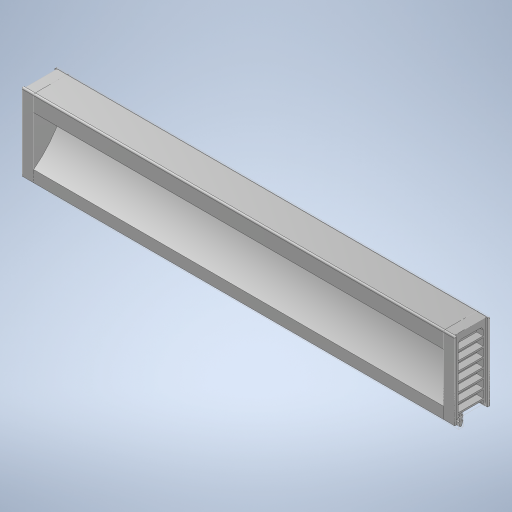
# Autodesk Inventor part: Hafele_alu_126_39
Saved by Autodesk Inventor 2024 (Build 280153000, 153)
## iProperties
RuleStatus: InUse
Created: 2019-10-04
Part Number: Hafele_alu_126_39
Material: Aluminum 6061
Document SubType Name: Modeling
Designer: RokasM
Density: 2.7 g/cm^3
Appearance: Anodized - Light Gray
AfterDocOpen0: LengthRule
Author: RokasM
Autodesk Inventor part; units mm, degrees
ref_plane "XZ Plane" through (0, 0, 0) normal (0, 1, 0) x (-1, 0, 0)
ref_plane "XY Plane" through (0, 0, 0) normal (0, 0, 1) x (1, 0, 0)
sketch "Sketch1" plane through (0, 0, 0) normal (1, 0, 0) x (0, 1, 0)
  line L0 (19.2576, 47.182) -> (19.2576, 36.782)
  line L1 (19.2576, 36.782) -> (21.0176, 36.782)
  arc A0 (24.8576, 45.482) -> (21.0176, 36.782) centre (44.137, 31.775) ccw
  line L2 (24.8576, 45.482) -> (38.8576, 45.482)
  line L3 (38.8576, 45.482) -> (38.8576, 34.7948)
  arc A1 (38.8223, 34.5717) -> (38.8576, 34.7948) centre (38.1341, 34.7948) ccw
  arc A2 (19.2576, 7.182) -> (38.8223, 34.5717) centre (-14.1874, 51.7546) ccw
  line L4 (19.2576, 7.182) -> (19.2576, 0.182)
  line L5 (19.2576, 0.182) -> (20.2576, 0.182)
  line L6 (20.2576, 0.182) -> (20.2576, 2.182)
  line L7 (20.2576, 2.182) -> (29.4376, 2.182)
  line L8 (29.4376, 2.182) -> (29.4376, -0.568)
  line L9 (29.4376, -0.568) -> (28.5076, -0.568)
  line L10 (28.5076, -0.568) -> (29.4376, -3.318)
  line L11 (29.4376, -3.318) -> (28.5076, -3.318)
  line L12 (28.5076, -3.318) -> (29.4376, -6.068)
  line L13 (29.4376, -6.068) -> (28.5076, -6.068)
  line L14 (28.5076, -6.068) -> (29.4376, -8.818)
  line L15 (29.4376, -8.818) -> (30.3776, -8.818)
  line L16 (30.3776, -8.818) -> (31.3076, -6.068)
  line L17 (31.3076, -6.068) -> (30.3776, -6.068)
  line L18 (30.3776, -6.068) -> (31.3076, -3.318)
  line L19 (31.3076, -3.318) -> (30.3776, -3.318)
  line L20 (30.3776, -3.318) -> (31.3076, -0.568)
  line L21 (31.3076, -0.568) -> (30.3776, -0.568)
  line L22 (30.3776, -0.568) -> (30.3776, 2.182)
  line L23 (30.3776, 2.182) -> (38.8576, 2.182)
  line L24 (38.8576, 2.182) -> (38.8576, 0.182)
  line L25 (38.8576, 0.182) -> (40.5576, 0.182)
  line L26 (40.5576, 0.182) -> (40.5576, 47.182)
  line L27 (40.5576, 47.182) -> (19.2576, 47.182)
  line L28 (21.6706, 3.882) -> (21.6706, 6.901)
  arc A3 (21.6706, 6.901) -> (38.8576, 29.7576) centre (-14.1874, 51.7546) ccw
  line L29 (38.8576, 29.7576) -> (38.8576, 3.882)
  line L30 (38.8576, 3.882) -> (21.6706, 3.882)
  point P0 (0, 0)
  dimension "d0" = 21.3
  dimension "d1" = 45
  dimension "d2" = 2
  dimension "d3" = 1
  dimension "d4" = 1.7
  dimension "d5" = 10.4
  dimension "d6" = 7
  dimension "d7" = 2.8
  dimension "d8" = 56
  dimension "d9" = 0.93
  dimension "d10" = 2.75
  dimension "d11" = 10.18
  dimension "d12" = 1.7
  dimension "d13" = 1.7
  dimension "d14" = 1.76
  dimension "d16" = 14
  dimension "d17" = 15.407
  dimension "d22" = 55.725
  dimension "d26" = 57.425
  dimension "d28" = 1.7
  dimension "d29" = 10.9103
  dimension "d30" = 2.413
  dimension "d31" = 1.7
  constraints: 62 end point, 10 horizontal, 9 vertical, 8 point on circle, 6 collinear, 6 vertical alignment, 5 equal length, 4 centre point, 4 parallel, 2 tangent, 1 concentric
  measures "d0" distance between parallel lines of L26 L0
  measures "d1" distance between parallel lines of L23 L27
  measures "d2" distance between parallel lines of L7 L5
  measures "d3" distance between parallel lines of L4 L6
  measures "d4" distance between parallel lines of L26 L24
  measures "d5" distance between parallel lines of L1 L27
  measures "d6" distance of L4.start L4.end
  measures "d7" distance of L16.end L13.end
  measures "d8" distance between parallel lines of L27 L15
  measures "d9" distance of L8.end L9.end
  measures "d10" distance between parallel lines of L11 L9
  measures "d11" distance between parallel lines of L8 L4
  measures "d12" distance between parallel lines of L2 L27
  measures "d13" distance between parallel lines of L26 L3
  measures "d14" distance of L0.end L1.end
  measures "d16" distance from line of L2.start L3
  measures "d17" distance from line of A0.centre L27
  measures "d22" radius of A2
  measures "d26" radius of A3
  measures "d28" distance between parallel lines of L26 L29
  measures "d29" distance from line of L2 A1.start
  measures "d30" distance between parallel lines of L4 L28
  measures "d31" distance between parallel lines of L7 L30
extrude "01_ex1" add sketch "Sketch1" along normal mid plane 250
fillet "01_fillet" radius 1.5 1 edges at (0, 38.8576, 29.7576)
fillet "01_fillet" radius 1 4 edges at (0, 21.0176, 36.782) (0, 19.2576, 47.182) (0, 38.8576, 45.482) (0, 40.5576, 47.182)
fillet "01_fillet" radius 0.5 6 edges at (0, 19.2576, 36.782) (0, 24.8576, 45.482) (0, 38.8576, 3.882) (0, 21.6706, 3.882) (0, 21.6706, 6.901) (0, 20.2576, 2.182)
ref_plane "wp_right" through (125, 0, 0) normal (1, 0, 0) x (0, 1, 0)
sketch "Sketch2" plane through (125, 0, 0) normal (1, 0, 0) x (0, 1, 0)
  line L0 (19.2576, 47.182) -> (40.5576, 47.182)
  line L1 (40.5576, 47.182) -> (40.5576, 0.182)
  line L2 (40.5576, 0.182) -> (19.2576, 0.182)
  line L3 (19.2576, 0.182) -> (19.2576, 47.182)
  line L4 (39.5576, 47.182) -> (20.2576, 47.182) projected
  line L5 (40.5576, 0.182) -> (40.5576, 46.182) projected
  point P0 (0, 0)
  dimension "d38" = 21.3
  dimension "d39" = 47
  constraints: 8 end point, 2 collinear, 2 parallel, 1 horizontal, 1 perpendicular
  measures "d38" distance between parallel lines of L1 L3
  measures "d39" distance between parallel lines of L2 L0
extrude "02_ex1" add sketch "Sketch2" along normal blind 7 separate body
sketch "Sketch3" plane through (132, 0, 0) normal (1, 0, 0) x (0, 0, -1)
  line L0 (-47.182, 20.2576) -> (-0.182, 20.2576)
  line L1 (-0.182, 20.2576) -> (-0.182, 39.1576)
  line L2 (-0.182, 39.1576) -> (-47.182, 39.1576)
  line L3 (-47.182, 39.1576) -> (-47.182, 20.2576)
  line L4 (-47.182, 19.2576) -> (-0.182, 19.2576) projected
  line L5 (-0.182, 19.2576) -> (-0.182, 40.5576) projected
  line L6 (-47.182, 40.5576) -> (-47.182, 19.2576) projected
  point P0 (0, 0)
  dimension "d42" = 18.9
  dimension "d43" = 1
  constraints: 8 end point, 2 collinear, 2 parallel, 1 horizontal, 1 perpendicular
  measures "d42" distance between parallel lines of L2 L0
  measures "d43" distance between parallel lines of L4 L0
extrude "02_ex2" cut sketch "Sketch3" against normal blind 1 contours L3 L2 L1 L0 bodies 2
sketch "Sketch4" plane through (131, 0, 0) normal (1, 0, 0) x (0, 0, -1)
  line L0 (-2.182, 39.1576) -> (-0.182, 39.1576)
  line L1 (-0.182, 39.1576) -> (-0.182, 20.2576)
  line L2 (-0.182, 20.2576) -> (-2.182, 20.2576)
  line L3 (-2.182, 20.2576) -> (-2.182, 39.1576)
  line L4 (-47.182, 39.1576) -> (-0.182, 39.1576) projected
  line L5 (-0.182, 20.2576) -> (-47.182, 20.2576) projected
  line L6 (-0.182, 39.1576) -> (-0.182, 20.2576) projected
  point P0 (0, 0)
  dimension "d46" = 2
  constraints: 8 end point, 3 collinear, 2 parallel, 1 horizontal, 1 perpendicular
  measures "d46" distance between parallel lines of L1 L3
extrude "02_ex3" cut sketch "Sketch4" against normal up to surface (6 mm away) bodies 2
sketch "Sketch5" plane through (131, 0, 0) normal (1, 0, 0) x (0, 0, -1)
  line L0 (-43.182, 22.2576) -> (-2.182, 22.2576)
  line L1 (-2.182, 22.2576) -> (-2.182, 37.5576)
  line L2 (-2.182, 37.5576) -> (-43.182, 37.5576)
  line L3 (-43.182, 37.5576) -> (-43.182, 22.2576)
  line L4 (-0.182, 20.2576) -> (-47.182, 20.2576) projected
  line L5 (-2.182, 20.2576) -> (-2.182, 39.1576) projected
  point P0 (0, 0)
  dimension "d49" = 41
  dimension "d50" = 15.3
  dimension "d51" = 2
  constraints: 8 end point, 2 parallel, 1 collinear, 1 horizontal, 1 perpendicular
  measures "d49" distance of L2.end L1.end
  measures "d50" distance of L1.end L0.end
  measures "d51" distance between parallel lines of L4 L0
extrude "02_ex4" cut sketch "Sketch5" against normal blind 4 bodies 2
sketch "Sketch6" plane through (127, 0, 0) normal (1, 0, 0) x (0, 0, -1)
  line L0 (-38.182, 22.2576) -> (-37.182, 22.2576)
  line L1 (-37.182, 22.2576) -> (-37.182, 37.5576)
  line L2 (-37.182, 37.5576) -> (-38.182, 37.5576)
  line L3 (-38.182, 37.5576) -> (-38.182, 22.2576)
  line L4 (-43.182, 22.2576) -> (-43.182, 37.5576) projected
  line L5 (-43.182, 37.5576) -> (-2.182, 37.5576) projected
  line L6 (-2.182, 22.2576) -> (-43.182, 22.2576) projected
  point P0 (0, 0)
  dimension "d54" = 1
  dimension "d55" = 5
  constraints: 8 end point, 2 collinear, 2 parallel, 1 horizontal, 1 perpendicular
  measures "d54" distance between parallel lines of L1 L3
  measures "d55" distance between parallel lines of L4 L3
extrude "02_ex5" add sketch "Sketch6" along normal up to surface (4 mm away) contours L3 L2 L1 L0 bodies 2
pattern_linear "02_pattern" count 7 spacing 5.5 along (0, 0, -1) of "02_ex5" bodies 2
sketch "Sketch7" plane through (125, 0, 0) normal (-1, 0, 0) x (0, 0, 1)
  arc A0 (37.5384, 21.1944) -> (45.2672, 24.7066) centre (31.775, 44.137) ccw projected
  arc A1 (45.2672, 24.7066) -> (45.482, 25.1173) centre (44.982, 25.1173) ccw projected
  line L0 (45.482, 37.8576) -> (45.482, 25.1173) projected
  arc A2 (45.482, 37.8576) -> (44.482, 38.8576) centre (44.482, 37.8576) ccw projected
  arc A3 (41.355, 23.0556) -> (44.982, 25.1166) centre (31.775, 44.137) ccw
  line L1 (44.982, 25.1166) -> (44.982, 37.8576)
  arc A4 (44.982, 37.8576) -> (44.482, 38.3576) centre (44.482, 37.8576) ccw
  line L2 (44.482, 38.3576) -> (44.482, 38.8576)
  line L3 (41.355, 23.0556) -> (41.5616, 22.601)
  point P0 (0, 0)
  dimension "d70" = 0.5
  dimension "d78" = 23.156
  constraints: 6 end point, 5 point on circle, 2 centre point, 1 line through centre, 1 vertical, 1 other
  measures "d70" distance between parallel lines of L0 L1
  measures "d78" radius of A3
extrude "02_ex6" add sketch "Sketch7" along normal blind 1 bodies 2
sketch "Sketch9" plane through (125, 0, 0) normal (-1, 0, 0) x (0, 0, 1)
  circle A0 centre (23.202, 37.3576) radius 1.5
  circle A1 centre (5.382, 23.1776) radius 1.5
  circle A2 centre (5.382, 37.3576) radius 1.5
  line L0 (0.182, 40.5576) -> (47.182, 40.5576) projected
  line L1 (2.182, 39.1576) -> (2.182, 20.2576) projected
  line L2 (47.182, 19.2576) -> (0.182, 19.2576) projected
  point P0 (0, 0)
  dimension "d83" = 3
  dimension "d84" = 3.2
  dimension "d85" = 3.2
  dimension "d86" = 3.2
  dimension "d87" = 3.2
  dimension "d88" = 21.02
  dimension "d89" = 3.92
  constraints: 3 centre point, 2 equal radius
  measures "d83" diameter of A0
  measures "d84" distance from line of L0 A0.centre
  measures "d85" distance from line of L0 A2.centre
  measures "d86" distance from line of L1 A2.centre
  measures "d87" distance from line of L1 A1.centre
  measures "d88" distance from line of L1 A0.centre
  measures "d89" distance from line of L2 A1.centre
extrude "02_ex7" add sketch "Sketch9" along normal blind 7 bodies 2
fillet "02_fillet" radius 2 2 edges at (129, 37.5576, 43.182) (129, 22.2576, 43.182)
fillet "02_fillet" radius 1 2 edges at (128.5, 19.2576, 47.182) (128.5, 40.5576, 47.182)
fillet "02_fillet" radius 0.5 2 edges at (128, 39.1576, 2.182) (128, 20.2576, 2.182)
mirror "02_mir" about plane through (0, 0, 0) normal (1, 0, 0) bodies 2
sketch "Sketch10" plane through (0, 0, 0) normal (1, 0, 0) x (0, 1, 0)
  line L0 (31.2576, 2.182) -> (31.2576, -9.818)
  line L1 (31.2576, -9.818) -> (28.5576, -9.818)
  line L2 (28.5576, -9.818) -> (28.5576, 2.182)
  line L3 (29.4376, -8.818) -> (30.3776, -8.818) projected
  line L4 (30.3776, 2.182) -> (38.8576, 2.182) projected
  line L5 (28.5576, 2.182) -> (20.2576, 2.182)
  line L6 (20.2576, 2.182) -> (20.2576, 0.182)
  line L7 (20.2576, 0.182) -> (19.2576, 0.182)
  line L8 (19.2576, 0.182) -> (19.2576, 47.182)
  line L9 (19.2576, 47.182) -> (40.5576, 47.182)
  line L10 (40.5576, 47.182) -> (40.5576, 0.182)
  line L11 (40.5576, 0.182) -> (38.8576, 0.182)
  line L12 (38.8576, 0.182) -> (38.8576, 2.182)
  line L13 (38.8576, 2.182) -> (31.2576, 2.182)
  line L14 (20.7576, 2.182) -> (29.4376, 2.182) projected
  line L15 (38.8576, 2.182) -> (38.8576, 0.182) projected
  line L16 (38.8576, 0.182) -> (40.5576, 0.182) projected
  line L17 (20.2576, 0.182) -> (20.2576, 1.682) projected
  line L18 (19.2576, 0.182) -> (20.2576, 0.182) projected
  line L19 (19.2576, 7.182) -> (19.2576, 0.182) projected
  line L20 (40.5576, 0.182) -> (40.5576, 46.182) projected
  line L21 (39.5576, 47.182) -> (20.2576, 47.182) projected
  point P0 (0, 0)
  point P1 (29.9076, -9.818)
  point P2 (29.9076, -8.818)
  dimension "d95" = 1
  dimension "d96" = 2.7
  constraints: 24 end point, 9 collinear, 2 midpoint, 1 parallel, 1 perpendicular, 1 vertical alignment
  measures "d95" distance between parallel lines of L3 L1
  measures "d96" distance between parallel lines of L2 L0
extrude "03_ex1" add sketch "Sketch10" along normal mid plane 250 separate body
sketch "Sketch13" plane through (125, 0, 0) normal (1, 0, 0) x (0, 0, -1)
  line L0 (-0.182, 19.2576) -> (-47.182, 19.2576)
  line L1 (-47.182, 19.2576) -> (-47.182, 40.5576)
  line L2 (-47.182, 40.5576) -> (-0.182, 40.5576)
  line L3 (-0.182, 40.5576) -> (-0.182, 38.8576)
  line L4 (-0.182, 38.8576) -> (-2.182, 38.8576)
  line L5 (-2.182, 38.8576) -> (-2.182, 20.2576)
  line L6 (-2.182, 20.2576) -> (-0.182, 20.2576)
  line L7 (-0.182, 20.2576) -> (-0.182, 19.2576)
  line L8 (-0.182, 19.2576) -> (-0.182, 20.2576) projected
  line L9 (-0.182, 20.2576) -> (-2.182, 20.2576) projected
  line L10 (-2.182, 20.2576) -> (-2.182, 28.5576) projected
  line L11 (-2.182, 38.8576) -> (-0.182, 38.8576) projected
  line L12 (-0.182, 38.8576) -> (-0.182, 40.5576) projected
  line L13 (-0.182, 40.5576) -> (-46.182, 40.5576) projected
  line L14 (-47.182, 19.2576) -> (-0.182, 19.2576) projected
  line L15 (-47.182, 40.5576) -> (-47.182, 19.2576) projected
  point P0 (0, 0)
  constraints: 16 end point, 8 collinear
extrude "04_ex1" add sketch "Sketch13" along normal blind 6 separate body
sketch "Sketch14" plane through (131, 0, 0) normal (1, 0, 0) x (0, 0, -1)
  line L0 (-47.182, 20.2576) -> (-0.182, 20.2576)
  line L1 (-0.182, 20.2576) -> (-0.182, 19.2576)
  line L2 (-0.182, 19.2576) -> (-47.182, 19.2576)
  line L3 (-47.182, 19.2576) -> (-47.182, 20.2576)
  line L4 (-47.182, 40.5576) -> (-0.182, 40.5576)
  line L5 (-0.182, 40.5576) -> (-0.182, 39.5576)
  line L6 (-0.182, 39.5576) -> (-47.182, 39.5576)
  line L7 (-47.182, 39.5576) -> (-47.182, 40.5576)
  line L8 (-47.182, 19.2576) -> (-0.182, 19.2576) projected
  line L9 (-47.182, 40.5576) -> (-47.182, 19.2576) projected
  line L10 (-0.182, 19.2576) -> (-0.182, 20.2576) projected
  line L11 (-0.182, 40.5576) -> (-47.182, 40.5576) projected
  point P0 (0, 0)
  dimension "d107" = 1
  constraints: 16 end point, 5 collinear, 4 parallel, 2 equal length, 2 horizontal, 2 perpendicular
  measures "d107" distance between parallel lines of L0 L2
extrude "04_ex2" add sketch "Sketch14" along normal blind 1 bodies 4
mirror "04_mir" about plane through (0, 0, 0) normal (1, 0, 0) bodies 4
equation "\"d26\" = d22 + d12"
equation "\"d28\" = d4"
equation "\"d31\" = d4"
equation "\"d32\" = Length"
equation "\"Length\" = 250"
equation "\"d37\" = 0.5 * Length"
